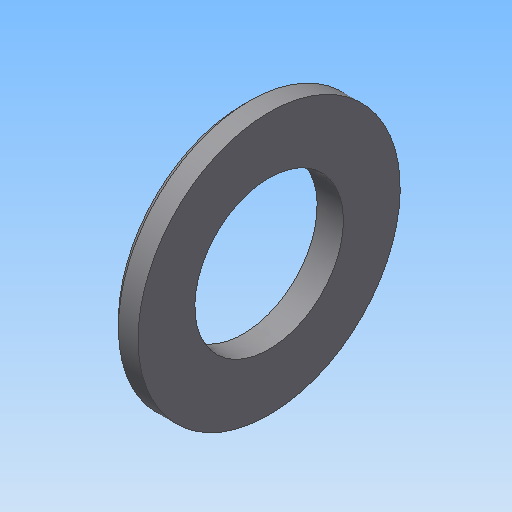
# Autodesk Inventor part: DIN 125-1 - B 17
Saved by Autodesk Inventor 2020.1 (Build 241239000, 239)
## iProperties
Comments: To add or edit properties for Autodesk Inventor files, use iProperties.
Shininess: 64.0
Length Units: 11269
Angle Units: 11279
Time Units: 11290
Mass Units: 11283
Length Display Precision: 3
Angle Display Precision: 2
Compacted: True
Alert: To add or edit properties for Autodesk Inventor files, use iProperties.
Library Location: C:\ap\Inventor 6\Content
Library: MyStandard
SubLibrary: DIN
Family: 162
Member: 310
Member Major Revision: 1
Member Minor Revision: 1
Created: 2003-02-27
Part Number: DIN 125-1 - B 17
Vendor: Autodesk Inc.
Document SubType Name: Modeling
Designer: Joe M
Description: Scheibe
Standard: DIN 125-1 B 17
Engineer: Joe M
Material: Generic
Density: 1 g/cm^3
Appearance: Default
Density: 0.0
Volumn: 0.0
Area: 0.0
PropertySet Name: Model Information
Control State: 0
Master: False
Checked Out: False
Author: Joe M
Autodesk Inventor part; units mm, degrees
ref_plane "YZ Plane" through (0, 0, 0) normal (1, 0, 0) x (0, 1, 0)
ref_plane "XZ Plane" through (0, 0, 0) normal (0, 1, 0) x (-1, 0, 0)
ref_plane "XY Plane" through (0, 0, 0) normal (0, 0, 1) x (1, 0, 0)
sketch "Skizze" plane through (0, 0, 0) normal (1, 0, 0) x (0, 1, 0)
  circle A0 centre (0, 0) radius 15
  circle A1 centre (0, 0) radius 8.5
  dimension "d0" = 17
  dimension "d1" = 30
  constraints: 2 centre point, 2 coincident
  measures "d0" diameter of A1
  measures "d1" diameter of A0
extrude "Körper" add sketch "Skizze" along normal blind 3
chamfer "Fase" distance 0.75 angle 45 1 edges at (0, -15, 0) measured on face at (2, 14.9514, -1.207)
equation "\"d0\" = SD1"
equation "\"d1\" = SD2"
equation "\"d2\" = SD"
equation "\"d4\" = PHH"
equation "\"d8\" = PHH"
equation "\"SD1\" = 17"
equation "\"SD2\" = 30"
equation "\"SD\" = 3"
equation "\"PHH\" = 0.75"
equation "\"FAWI\" = 45deg"
equation "\"NND\" = 16"
body "Solid1"
